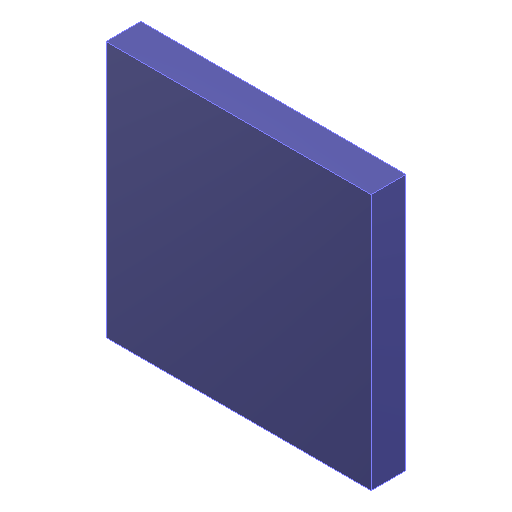
# Autodesk Inventor part: 1751248
Saved by Autodesk Inventor 2022 (Build 260153000, 153)
## iProperties
Created: 2022-01-18
Part Number: 1751248
Material: Generisch
Document SubType Name: Modeling
Designer: diederichbenedict
Density: 1 g/cm^3
Appearance: 1751248, 1751248
Author: diederichbenedict
Autodesk Inventor part; units mm, degrees
ref_plane "YZ Plane" through (0, 0, 0) normal (1, 0, 0) x (0, 1, 0)
ref_plane "XZ Plane" through (0, 0, 0) normal (0, 1, 0) x (-1, 0, 0)
ref_plane "XY Plane" through (0, 0, 0) normal (0, 0, 1) x (1, 0, 0)
sketch "1751248, 1751248_1" plane through (0, 0, 0) normal (0, 0, 1) x (1, 0, 0)
  line L0 (-3.8008, 3.7008) -> (3.8008, 3.7008)
  line L1 (3.8008, 3.7008) -> (3.8008, -3.65)
  line L2 (3.8008, -3.65) -> (-3.8008, -3.65)
  line L3 (-3.8008, -3.65) -> (-3.8008, 3.7008)
  constraints: 8 end point
extrude "Extrusion1" add sketch "1751248, 1751248_1" along normal blind 1
